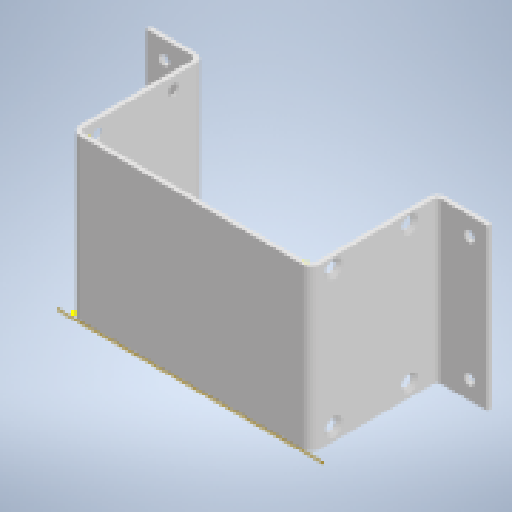
# Autodesk Inventor part: Top
Saved by Autodesk Inventor 2024 (Build 280153000, 153)
## iProperties
Created: 2025-10-29
Part Number: Top
Material: 일반
Document SubType Name: Sheet Metal
Designer: alexi
Density: 1 g/cm^3
Appearance: 기본값
Sheet Metal Rule: 기본값
Author: alexi
Autodesk Inventor part; units mm, degrees
ref_plane "YZ Plane" through (0, 0, 0) normal (1, 0, 0) x (0, 1, 0)
ref_plane "XZ Plane" through (0, 0, 0) normal (0, 1, 0) x (-1, 0, 0)
ref_plane "XY Plane" through (0, 0, 0) normal (0, 0, 1) x (1, 0, 0)
ref_plane "작업 평면1" through (0, 0, 0) normal (0, 0, 1) x (1, 0, 0)
sketch "스케치1" plane through (0, 0, 0) normal (0, 0, 1) x (1, 0, 0)
  line L0 (80, 11.5982) -> (80.0982, 11.5982) projected
  line L1 (80.0982, 41.5982) -> (80, 41.5982) projected
  line L2 (0, 41.5982) -> (-0.0982, 41.5982) projected
  line L3 (4.8929, 0.1982) -> (3.2829, 0.1982)
  line L4 (3.2829, 0.1982) -> (3.2829, 52.9982)
  line L5 (3.2829, 52.9982) -> (4.8929, 52.9982)
  line L6 (4.8929, 52.9982) -> (4.8929, 0.1982)
  line L7 (3.2829, 0.1982) -> (-0.2171, 0.1982)
  line L8 (-0.2171, 0.1982) -> (-0.2171, 52.9982)
  line L9 (-0.2171, 52.9982) -> (3.2829, 52.9982)
  line L10 (3.2829, 52.9982) -> (3.2829, 0.1982)
  line L11 (-0.2171, 0.1982) -> (-37.1171, 0.1982)
  line L12 (-37.1171, 0.1982) -> (-37.1171, 52.9982)
  line L13 (-37.1171, 52.9982) -> (-0.2171, 52.9982)
  line L14 (-0.2171, 52.9982) -> (-0.2171, 0.1982)
  line L15 (4.8929, 52.9982) -> (4.8929, 0.1982)
  line L16 (75.1071, 0.1982) -> (76.7171, 0.1982)
  line L17 (76.7171, 0.1982) -> (76.7171, 52.9982)
  line L18 (76.7171, 52.9982) -> (75.1071, 52.9982)
  line L19 (75.1071, 52.9982) -> (75.1071, 0.1982)
  line L20 (76.7171, 0.1982) -> (80.2171, 0.1982)
  line L21 (80.2171, 0.1982) -> (80.2171, 52.9982)
  line L22 (80.2171, 52.9982) -> (76.7171, 52.9982)
  line L23 (76.7171, 52.9982) -> (76.7171, 0.1982)
  line L24 (80.2171, 0.1982) -> (117.1171, 0.1982)
  line L25 (117.1171, 0.1982) -> (117.1171, 52.9982)
  line L26 (117.1171, 52.9982) -> (80.2171, 52.9982)
  line L27 (80.2171, 52.9982) -> (80.2171, 0.1982)
  line L28 (4.8929, 0.1982) -> (75.1071, 0.1982)
  line L29 (75.1071, 52.9982) -> (4.8929, 52.9982)
  line L30 (-37.1171, 0.1982) -> (-40.6171, 0.1982)
  line L31 (-40.6171, 0.1982) -> (-40.6171, 52.9982)
  line L32 (-40.6171, 52.9982) -> (-37.1171, 52.9982)
  line L33 (-37.1171, 52.9982) -> (-37.1171, 0.1982)
  line L34 (-40.6171, 0.1982) -> (-55.6171, 0.1982)
  line L35 (-55.6171, 0.1982) -> (-55.6171, 52.9982)
  line L36 (-55.6171, 52.9982) -> (-40.6171, 52.9982)
  line L37 (-40.6171, 52.9982) -> (-40.6171, 0.1982)
  line L38 (117.1171, 0.1982) -> (120.6171, 0.1982)
  line L39 (120.6171, 0.1982) -> (120.6171, 52.9982)
  line L40 (120.6171, 52.9982) -> (117.1171, 52.9982)
  line L41 (117.1171, 52.9982) -> (117.1171, 0.1982)
  line L42 (120.6171, 0.1982) -> (135.6171, 0.1982)
  line L43 (135.6171, 0.1982) -> (135.6171, 52.9982)
  line L44 (135.6171, 52.9982) -> (120.6171, 52.9982)
  line L45 (120.6171, 52.9982) -> (120.6171, 0.1982)
  line L46 (2, 1.5982) -> (78, 1.5982) projected
  line L47 (78, 1.5982) -> (78, 11.0982) projected
  line L48 (78, 11.0982) -> (75, 11.0982) projected
  line L49 (75, 11.0982) -> (75, 11.5982) projected
  line L50 (75, 11.5982) -> (75.1071, 11.5982) projected
  line L51 (75.1071, 11.5982) -> (75.1071, 41.5982) projected
  line L52 (75.1071, 41.5982) -> (75, 41.5982) projected
  line L53 (75, 41.5982) -> (75, 42.0982) projected
  line L54 (75, 42.0982) -> (78, 42.0982) projected
  line L55 (78, 42.0982) -> (78, 51.5982) projected
  line L56 (78, 51.5982) -> (2, 51.5982) projected
  line L57 (2, 51.5982) -> (2, 42.0982) projected
  line L58 (2, 42.0982) -> (5, 42.0982) projected
  line L59 (5, 42.0982) -> (5, 41.5982) projected
  line L60 (5, 41.5982) -> (4.8929, 41.5982) projected
  line L61 (4.8929, 41.5982) -> (4.8929, 11.5982) projected
  line L62 (4.8929, 11.5982) -> (5, 11.5982) projected
  line L63 (5, 11.5982) -> (5, 11.0982) projected
  line L64 (5, 11.0982) -> (2, 11.0982) projected
  line L65 (2, 11.0982) -> (2, 1.5982) projected
  line L66 (2, -1.4018) -> (78, -1.4018) projected
  line L67 (78, 0.0982) -> (78, -1.4018) projected
  line L68 (2, 0.0982) -> (78, 0.0982) projected
  line L69 (2, 0.0982) -> (2, -1.4018) projected
  line L70 (78, 54.5982) -> (2, 54.5982) projected
  line L71 (2, 53.0982) -> (2, 54.5982) projected
  line L72 (78, 53.0982) -> (2, 53.0982) projected
  line L73 (78, 53.0982) -> (78, 54.5982) projected
  point P0 (0, 0)
  point P1 (117.1171, 52.9982)
  dimension "d98" = 0.1
  dimension "d0" = 1.61
  dimension "d1" = 3.5
  dimension "d2" = 36.9
  dimension "d3" = 1.61
  dimension "d4" = 3.5
  dimension "d5" = 36.9
  dimension "d33" = 3.5
  dimension "d34" = 3.5
  dimension "d35" = 15
  dimension "d36" = 15
  dimension "d97" = 0.1
  constraints: 78 end point, 19 parallel, 8 horizontal, 8 perpendicular, 5 point on line, 3 collinear, 2 vertical, 15 other
  measures "d0" distance of L5.end L4.end
  measures "d1" distance of L8.end L10.start
  measures "d2" distance of L12.end L13.end
  measures "d3" distance of L18.end L17.end
  measures "d4" distance of L21.end L23.start
  measures "d5" distance of L21.end L25.end
  measures "d33" distance of L12.end L31.end
  measures "d34" distance of L39.end L40.end
  measures "d35" distance of L35.end L36.end
  measures "d36" distance of L43.end L44.end
extrude "판1" add sketch "스케치1" against normal blind 1.5 contours L3 L4 L46 L6 | L6 L46 L19 L28 | L7 L8 L9 L4 L56 L57 L58 L64 L65 L46 | L46 L4 L64 L6 | L6 L64 L63 L62 L60 L59 L58 L56 L19 L54 L53 L52 L50 L49 L48 L46 | L19 L46 L17 L16 | L46 L65 L64 L4 | L11 L12 L13 L8 | L64 L4 L58 L6 | L6 L62 L63 L64 | L19 L48 L17 L46 | L17 L46 L47 L48 L54 L55 L56 L22 L21 L20 | L30 L31 L32 L12 | L48 L49 L50 L19 | L19 L54 L17 L48 | L17 L48 L47 L46 | L21 L26 L25 L24 | L58 L57 L56 L4 | L4 L56 L6 L58 | L5 L6 L56 L4 | L34 L35 L36 L31 | L6 L58 L59 L60 | L25 L40 L39 L38 | L29 L19 L56 L6 | L52 L53 L54 L19 | L54 L19 L56 L17 | L17 L56 L55 L54 | L17 L56 L19 L18 | L39 L44 L43 L42
sketch "스케치2" plane through (0, 0, -1.5) normal (0, 0, -1) x (-1, 0, 0)
  line L0 (-4.8929, 52.9982) -> (-4.8929, 0.1982) projected
  line L1 (-3.2829, 0.1982) -> (-3.2829, 52.9982) projected
  line L2 (-75.1071, 52.9982) -> (-75.1071, 0.1982) projected
  line L3 (-76.7171, 52.9982) -> (-76.7171, 0.1982) projected
  point P0 (0, 0)
  point P1 (-4.8929, 0.1982)
  constraints: 1 other
fold "접기3" angle 90 bend radius 1.5 thickness 1.5 k factor 0.44 line from (-37.1171, 0.1982, 0) to (-37.1171, 52.9982, 0) line at bend start moving side (-1, 0, 0) folds toward (0, 0, 1)
fold "접기4" angle 90 bend radius 1.5 thickness 1.5 k factor 0.44 line from (117.1171, 0.1982, 0) to (117.1171, 52.9982, 0) line at bend start moving side (1, 0, 0) folds toward (0, 0, 1)
fold "접기5" angle 90 bend radius 1.5 thickness 1.5 k factor 0.44 line from (76.7171, 52.9982, -1.5) to (76.7171, 0.1982, -1.5) line at bend start moving side (1, 0, 0) folds toward (0, 0, -1)
fold "접기6" angle 90 bend radius 1.5 thickness 1.5 k factor 0.44 line from (3.2829, 0.1982, -1.5) to (3.2829, 52.9982, -1.5) line at bend start moving side (-1, 0, 0) folds toward (0, 0, -1)
sketch "스케치5" plane through (0.2829, 52.9982, -40.0071) normal (-1, 0, 0) x (0, 0, 1)
  circle A0 centre (32.5071, -3.9) radius 1.2295 projected
  circle A1 centre (7.5071, -3.9) radius 1.2295 projected
  circle A2 centre (7.5071, -48.9) radius 1.2295 projected
  circle A3 centre (32.5071, -48.9) radius 1.2295 projected
  point P0 (40.0071, -52.9982)
  constraints: 4 coincident
hole "구멍3" at (0.2829, 49.0982, -7.5) at (0.2829, 49.0982, -32.5) at (0.2829, 4.0982, -32.5) at (0.2829, 4.0982, -7.5) direction (1, 0, 0) diameter 3.4 depth 1.5 tip angle 118 countersink diameter 5.8 countersink angle 90
sketch "스케치6" plane through (79.7171, 0.1982, -3) normal (1, 0, 0) x (0, 0, -1)
  circle A0 centre (4.5, 3.9) radius 1.2295 projected
  circle A1 centre (29.5, 3.9) radius 1.2295 projected
  circle A2 centre (29.5, 48.9) radius 1.2295 projected
  circle A3 centre (4.5, 48.9) radius 1.2295 projected
  point P0 (-3, -0.1982)
  constraints: 7 coincident
hole "구멍4" at (79.7171, 4.0982, -7.5) at (79.7171, 4.0982, -32.5) at (79.7171, 49.0982, -32.5) at (79.7171, 49.0982, -7.5) at (79.7171, 4.0982, -7.5) at (79.7171, 4.0982, -32.5) at (79.7171, 49.0982, -32.5) direction (-1, 0, 0) diameter 3.4 depth 1.5 tip angle 118 countersink diameter 5.8 countersink angle 90
sketch "스케치7" plane through (-16.3242, 52.9982, -41.5071) normal (0, 0, 1) x (1, 0, 0)
  line L0 (0, 0) -> (0, -52.8) projected
  line L1 (15.1071, 0) -> (0, 0) projected
  line L2 (0, -52.8) -> (15.1071, -52.8) projected
  point P0 (16.3242, -52.9982)
  point P1 (6, -6)
  point P2 (6, -46.8)
  dimension "d75" = 6
  dimension "d76" = 6
  dimension "d77" = 6
  dimension "d78" = 6
  measures "d75" distance from line of L0 point (6, -6)
  measures "d76" distance from line of L1 point (6, -6)
  measures "d77" distance from line of L2 point (6, -46.8)
  measures "d78" distance from line of L0 point (6, -46.8)
sketch "스케치8" plane through (81.2171, 0.1982, -41.5071) normal (0, 0, 1) x (1, 0, 0)
  line L0 (15.1071, 0) -> (15.1071, 52.8) projected
  line L1 (15.1071, 52.8) -> (0, 52.8) projected
  line L2 (0, 0) -> (15.1071, 0) projected
  point P0 (-81.2171, -0.1982)
  point P1 (9.1071, 46.8)
  point P2 (9.1071, 6)
  dimension "d79" = 6
  dimension "d80" = 6
  dimension "d81" = 6
  dimension "d82" = 6
  measures "d79" distance from line of L0 point (9.107, 46.8)
  measures "d80" distance from line of L1 point (9.107, 46.8)
  measures "d81" distance from line of L2 point (9.107, 6)
  measures "d82" distance from line of L0 point (9.107, 6)
hole "구멍5" at (-10.3242, 46.9982, -41.5071) at (-10.3242, 6.1982, -41.5071) direction (0, 0, -1) diameter 3.4 depth 1.5 tip angle 118
hole "구멍6" at (90.3242, 46.9982, -41.5071) at (90.3242, 6.1982, -41.5071) direction (0, 0, -1) diameter 3.4 depth 1.5 tip angle 118
equation "\"d1\" = d4"
equation "\"d2\" = d5"
equation "\"d33\" = d4"
equation "\"d34\" = d4"
equation "\"d37\" = BendReliefWidth"
equation "\"d38\" = BendReliefDepth"
equation "\"d39\" = MinimumRemnant"
equation "\"d40\" = TransitionRadius"
equation "\"d43\" = BendReliefWidth"
equation "\"d44\" = BendReliefDepth"
equation "\"d45\" = MinimumRemnant"
equation "\"d46\" = TransitionRadius"
equation "\"d49\" = BendReliefWidth"
equation "\"d50\" = BendReliefDepth"
equation "\"d51\" = MinimumRemnant"
equation "\"d52\" = TransitionRadius"
equation "\"d55\" = BendReliefWidth"
equation "\"d56\" = BendReliefDepth"
equation "\"d57\" = MinimumRemnant"
equation "\"d58\" = TransitionRadius"
equation "\"TransitionRadius\" = BendRadius"
equation "\"BendReliefWidth\" = 1.5"
equation "\"BendReliefDepth\" = 0.75"
equation "\"MinimumRemnant\" = 3"
equation "\"BendRadius\" = 1.5"
